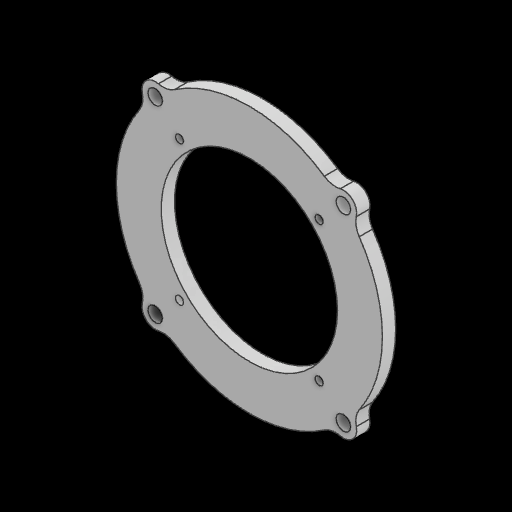
# Autodesk Inventor part: CimCoderMount
Saved by Autodesk Inventor 2025.2 (Build 292293000, 293)
## iProperties
Created: 2026-01-26
Part Number: CimCoderMount
Material: Generic
Document SubType Name: Sheet Metal
Designer: valer
Density: 1 g/cm^3
Appearance: Default
Sheet Metal Rule: Default
Author: valer
Autodesk Inventor part; units mm, degrees
ref_plane "YZ Plane" through (0, 0, 0) normal (1, 0, 0) x (0, 1, 0)
ref_plane "XZ Plane" through (0, 0, 0) normal (0, 1, 0) x (-1, 0, 0)
ref_plane "XY Plane" through (0, 0, 0) normal (0, 0, 1) x (1, 0, 0)
sketch "Base" plane through (0, 0, 0) normal (0, 0, 1) x (1, 0, 0)
  line L0 (-56, 0) -> (56, 0)
  line L1 (0, -56) -> (0, 56) construction
  circle A0 centre (0, 0) radius 40
  line L2 (0, 0) -> (28.2843, 28.2843) construction
  circle A1 centre (28.2843, 28.2843) radius 2.2
  circle A2 centre (-28.2843, 28.2843) radius 2.2
  circle A3 centre (28.2843, -28.2843) radius 2.2
  circle A4 centre (-28.2843, -28.2843) radius 2.2
  circle A5 centre (28.2843, 28.2843) radius 4
  circle A6 centre (-28.2843, 28.2843) radius 4
  circle A7 centre (28.2843, -28.2843) radius 4
  circle A8 centre (-28.2843, -28.2843) radius 4
  circle A9 centre (0, 0) radius 12.2174 construction
  spline S0 degree 3 number of poles 906
  spline S1 degree 3 number of poles 906
  spline S2 degree 3 number of poles 906
  spline S3 degree 3 number of poles 906
  spline S4 degree 2 poles (23.8703, -1.5488) (24.7501, -1.6971) (25.0615, -2.5332) (25.373, -3.3693) (24.8047, -4.057) (24.2364, -4.7448) (23.3566, -4.5965) (22.4768, -4.4482) (22.1653, -3.6122) (21.8538, -2.7761) (22.4222, -2.0883) (22.9905, -1.4006) (23.8703, -1.5488) (24.7501, -1.6971) (25.0615, -2.5332) (25.373, -3.3693) (24.8047, -4.057) (24.2364, -4.7448) (23.3566, -4.5965) (22.4768, -4.4482) (22.1653, -3.6122) (21.8538, -2.7761) (22.4222, -2.0883) (22.9905, -1.4006) (23.8703, -1.5488) (24.7501, -1.6971) (25.0615, -2.5332) (25.373, -3.3693) (24.8047, -4.057) (24.2364, -4.7448) (23.3566, -4.5965) (22.4768, -4.4482) (22.1653, -3.6122) (21.8538, -2.7761) (22.4222, -2.0883) (22.9905, -1.4006) (23.8703, -1.5488) (24.7501, -1.6971) (25.0615, -2.5332) (25.373, -3.3693) (24.8047, -4.057) (24.2364, -4.7448) (23.3566, -4.5965) (22.4768, -4.4482) (22.1653, -3.6122) (21.8538, -2.7761) (22.4222, -2.0883) (22.9905, -1.4006) (23.8703, -1.5488) (24.7501, -1.6971) (25.0615, -2.5332) (25.373, -3.3693) (24.8047, -4.057) (24.2364, -4.7448) (23.3566, -4.5965) (22.4768, -4.4482) (22.1653, -3.6122) (21.8538, -2.7761) (22.4222, -2.0883) (22.9905, -1.4006) (23.8703, -1.5488) (24.7501, -1.6971) (25.0615, -2.5332) (25.373, -3.3693) (24.8047, -4.057) (24.2364, -4.7448) (23.3566, -4.5965) (22.4768, -4.4482) (22.1653, -3.6122) (21.8538, -2.7761) (22.4222, -2.0883) (22.9905, -1.4006) (23.8703, -1.5488) (24.7501, -1.6971) (25.0615, -2.5332) (25.373, -3.3693) (24.8047, -4.057) (24.2364, -4.7448) (23.3566, -4.5965) (22.4768, -4.4482) (22.1653, -3.6122) (21.8538, -2.7761) (22.4222, -2.0883) (22.9905, -1.4006) (23.8703, -1.5488) (24.7501, -1.6971) (25.0615, -2.5332) (25.373, -3.3693) (24.8047, -4.057) (24.2364, -4.7448) (23.3566, -4.5965) (22.4768, -4.4482) (22.1653, -3.6122) (21.8538, -2.7761) (22.4222, -2.0883) (22.9905, -1.4006) (23.8703, -1.5488) (24.7501, -1.6971) (25.0615, -2.5332) (25.373, -3.3693) (24.8047, -4.057) (24.2364, -4.7448) (23.3566, -4.5965) (22.4768, -4.4482) (22.1653, -3.6122) (21.8538, -2.7761) (22.4222, -2.0883) (22.9905, -1.4006) (23.8703, -1.5488) (24.7501, -1.6971) (25.0615, -2.5332) (25.373, -3.3693) (24.8047, -4.057) (24.2364, -4.7448) (23.3566, -4.5965) (22.4768, -4.4482) (22.1653, -3.6122) (21.8538, -2.7761) (22.4222, -2.0883) (22.9905, -1.4006) (23.8703, -1.5488) (24.7501, -1.6971) (25.0615, -2.5332) (25.373, -3.3693) (24.8047, -4.057) (24.2364, -4.7448) (23.3566, -4.5965) (22.4768, -4.4482) (22.1653, -3.6122) (21.8538, -2.7761) (22.4222, -2.0883) (22.9905, -1.4006) (23.8703, -1.5488) (24.7501, -1.6971) (25.0615, -2.5332) (25.373, -3.3693) (24.8047, -4.057) (24.2364, -4.7448) (23.3566, -4.5965) (22.4768, -4.4482) (22.1653, -3.6122) (21.8538, -2.7761) (22.4222, -2.0883) (22.9905, -1.4006) (23.8703, -1.5488) (24.7501, -1.6971) (25.0615, -2.5332) (25.373, -3.3693) (24.8047, -4.057) (24.2364, -4.7448) (23.3566, -4.5965) (22.4768, -4.4482) (22.1653, -3.6122) (21.8538, -2.7761) (22.4222, -2.0883) (22.9905, -1.4006) (23.8703, -1.5488) (24.7501, -1.6971) (25.0615, -2.5332) (25.373, -3.3693) (24.8047, -4.057) (24.2364, -4.7448) (23.3566, -4.5965) (22.4768, -4.4482) (22.1653, -3.6122) (21.8538, -2.7761) (22.4222, -2.0883) (22.9905, -1.4006) (23.8703, -1.5488) (24.7501, -1.6971) (25.0615, -2.5332) (25.373, -3.3693) (24.8047, -4.057) (24.2364, -4.7448) (23.3566, -4.5965) (22.4768, -4.4482) (22.1653, -3.6122) (21.8538, -2.7761) (22.4222, -2.0883) (22.9905, -1.4006) (23.8703, -1.5488) (24.7501, -1.6971) (25.0615, -2.5332) (25.373, -3.3693) (24.8047, -4.057) (24.2364, -4.7448) (23.3566, -4.5965) (22.4768, -4.4482) (22.1653, -3.6122) (21.8538, -2.7761) (22.4222, -2.0883) (22.9905, -1.4006) (23.8703, -1.5488) (24.7501, -1.6971) (25.0615, -2.5332) (25.373, -3.3693) (24.8047, -4.057) (24.2364, -4.7448) (23.3566, -4.5965) (22.4768, -4.4482) (22.1653, -3.6122) (21.8538, -2.7761) (22.4222, -2.0883) (22.9905, -1.4006) (23.8703, -1.5488) (24.7501, -1.6971) (25.0615, -2.5332) (25.373, -3.3693) (24.8047, -4.057) (24.2364, -4.7448) (23.3566, -4.5965) (22.4768, -4.4482) (22.1653, -3.6122) (21.8538, -2.7761) (22.4222, -2.0883) (22.9905, -1.4006) (23.8703, -1.5488) (24.7501, -1.6971) (25.0615, -2.5332) (25.373, -3.3693) (24.8047, -4.057) (24.2364, -4.7448) (23.3566, -4.5965) (22.4768, -4.4482) (22.1653, -3.6122) (21.8538, -2.7761) (22.4222, -2.0883) (22.9905, -1.4006) (23.8703, -1.5488) (24.7501, -1.6971) (25.0615, -2.5332) (25.373, -3.3693) (24.8047, -4.057) (24.2364, -4.7448) (23.3566, -4.5965) (22.4768, -4.4482) (22.1653, -3.6122) (21.8538, -2.7761) (22.4222, -2.0883) (22.9905, -1.4006) (23.8703, -1.5488) (24.7501, -1.6971) (25.0615, -2.5332) (25.373, -3.3693) (24.8047, -4.057) (24.2364, -4.7448) (23.3566, -4.5965) (22.4768, -4.4482) (22.1653, -3.6122) (21.8538, -2.7761) (22.4222, -2.0883) (22.9905, -1.4006) (23.8703, -1.5488) (24.7501, -1.6971) (25.0615, -2.5332) (25.373, -3.3693) (24.8047, -4.057) (24.2364, -4.7448) (23.3566, -4.5965) (22.4768, -4.4482) (22.1653, -3.6122) (21.8538, -2.7761) (22.4222, -2.0883) (22.9905, -1.4006) (23.8703, -1.5488) (24.7501, -1.6971) (25.0615, -2.5332) (25.373, -3.3693) (24.8047, -4.057) (24.2364, -4.7448) (23.3566, -4.5965) (22.4768, -4.4482) (22.1653, -3.6122) (21.8538, -2.7761) (22.4222, -2.0883) (22.9905, -1.4006) (23.8703, -1.5488) (24.7501, -1.6971) (25.0615, -2.5332) (25.373, -3.3693) (24.8047, -4.057) (24.2364, -4.7448) (23.3566, -4.5965) (22.4768, -4.4482) (22.1653, -3.6122) (21.8538, -2.7761) (22.4222, -2.0883) (22.9905, -1.4006) (23.8703, -1.5488) (24.7501, -1.6971) (25.0615, -2.5332) (25.373, -3.3693) (24.8047, -4.057) (24.2364, -4.7448) (23.3566, -4.5965) (22.4768, -4.4482) (22.1653, -3.6122) (21.8538, -2.7761) (22.4222, -2.0883) (22.9905, -1.4006) (23.8703, -1.5488) (24.7501, -1.6971) (25.0615, -2.5332) (25.373, -3.3693) (24.8047, -4.057) (24.2364, -4.7448) (23.3566, -4.5965) (22.4768, -4.4482) (22.1653, -3.6122) (21.8538, -2.7761) (22.4222, -2.0883) (22.9905, -1.4006) (23.8703, -1.5488) (24.7501, -1.6971) (25.0615, -2.5332) (25.373, -3.3693) (24.8047, -4.057) (24.2364, -4.7448) (23.3566, -4.5965) (22.4768, -4.4482) (22.1653, -3.6122) (21.8538, -2.7761) (22.4222, -2.0883) (22.9905, -1.4006) (23.8703, -1.5488) (24.7501, -1.6971) (25.0615, -2.5332) (25.373, -3.3693) (24.8047, -4.057) (24.2364, -4.7448) (23.3566, -4.5965) (22.4768, -4.4482) (22.1653, -3.6122) (21.8538, -2.7761) (22.4222, -2.0883) (22.9905, -1.4006) (23.8703, -1.5488) (24.7501, -1.6971) (25.0615, -2.5332) (25.1147, -2.6758) (25.139, -2.8261) knots 0.016667 0.016667 0.016667 0.022222 0.022222 0.027778 0.027778 0.033333 0.033333 0.038889 0.038889 0.044444 0.044444 0.05 0.05 0.055556 0.055556 0.061111 0.061111 0.066667 0.066667 0.072222 0.072222 0.077778 0.077778 0.083333 0.083333 0.088889 0.088889 0.094444 0.094444 0.1 0.1 0.105556 0.105556 0.111111 0.111111 0.116667 0.116667 0.122222 0.122222 0.127778 0.127778 0.133333 0.133333 0.138889 0.138889 0.144444 0.144444 0.15 0.15 0.155556 0.155556 0.161111 0.161111 0.166667 0.166667 0.172222 0.172222 0.177778 0.177778 0.183333 0.183333 0.188889 0.188889 0.194444 0.194444 0.2 0.2 0.205556 0.205556 0.211111 0.211111 0.216667 0.216667 0.222222 0.222222 0.227778 0.227778 0.233333 0.233333 0.238889 0.238889 0.244444 0.244444 0.25 0.25 0.255556 0.255556 0.261111 0.261111 0.266667 0.266667 0.272222 0.272222 0.277778 0.277778 0.283333 0.283333 0.288889 0.288889 0.294444 0.294444 0.3 0.3 0.305556 0.305556 0.311111 0.311111 0.316667 0.316667 0.322222 0.322222 0.327778 0.327778 0.333333 0.333333 0.338889 0.338889 0.344444 0.344444 0.35 0.35 0.355556 0.355556 0.361111 0.361111 0.366667 0.366667 0.372222 0.372222 0.377778 0.377778 0.383333 0.383333 0.388889 0.388889 0.394444 0.394444 0.4 0.4 0.405556 0.405556 0.411111 0.411111 0.416667 0.416667 0.422222 0.422222 0.427778 0.427778 0.433333 0.433333 0.438889 0.438889 0.444444 0.444444 0.45 0.45 0.455556 0.455556 0.461111 0.461111 0.466667 0.466667 0.472222 0.472222 0.477778 0.477778 0.483333 0.483333 0.488889 0.488889 0.494444 0.494444 0.5 0.5 0.505556 0.505556 0.511111 0.511111 0.516667 0.516667 0.522222 0.522222 0.527778 0.527778 0.533333 0.533333 0.538889 0.538889 0.544444 0.544444 0.55 0.55 0.555556 0.555556 0.561111 0.561111 0.566667 0.566667 0.572222 0.572222 0.577778 0.577778 0.583333 0.583333 0.588889 0.588889 0.594444 0.594444 0.6 0.6 0.605556 0.605556 0.611111 0.611111 0.616667 0.616667 0.622222 0.622222 0.627778 0.627778 0.633333 0.633333 0.638889 0.638889 0.644444 0.644444 0.65 0.65 0.655556 0.655556 0.661111 0.661111 0.666667 0.666667 0.672222 0.672222 0.677778 0.677778 0.683333 0.683333 0.688889 0.688889 0.694444 0.694444 0.7 0.7 0.705556 0.705556 0.711111 0.711111 0.716667 0.716667 0.722222 0.722222 0.727778 0.727778 0.733333 0.733333 0.738889 0.738889 0.744444 0.744444 0.75 0.75 0.755556 0.755556 0.761111 0.761111 0.766667 0.766667 0.772222 0.772222 0.777778 0.777778 0.783333 0.783333 0.788889 0.788889 0.794444 0.794444 0.8 0.8 0.805556 0.805556 0.811111 0.811111 0.816667 0.816667 0.822222 0.822222 0.827778 0.827778 0.833333 0.833333 0.838889 0.838889 0.844444 0.844444 0.85 0.85 0.855556 0.855556 0.861111 0.861111 0.866667 0.866667 0.872222 0.872222 0.877778 0.877778 0.883333 0.883333 0.888889 0.888889 0.894444 0.894444 0.9 0.9 0.905556 0.905556 0.911111 0.911111 0.916667 0.916667 0.922222 0.922222 0.927778 0.927778 0.933333 0.933333 0.938889 0.938889 0.944444 0.944444 0.95 0.95 0.955556 0.955556 0.956622 0.956622 0.956622 weights 1 0.866025 1 0.866025 1 0.866025 1 0.866025 1 0.866025 1 0.866025 1 0.866025 1 0.866025 1 0.866025 1 0.866025 1 0.866025 1 0.866025 1 0.866025 1 0.866025 1 0.866025 1 0.866025 1 0.866025 1 0.866025 1 0.866025 1 0.866025 1 0.866025 1 0.866025 1 0.866025 1 0.866025 1 0.866025 1 0.866025 1 0.866025 1 0.866025 1 0.866025 1 0.866025 1 0.866025 1 0.866025 1 0.866025 1 0.866025 1 0.866025 1 0.866025 1 0.866025 1 0.866025 1 0.866025 1 0.866025 1 0.866025 1 0.866025 1 0.866025 1 0.866025 1 0.866025 1 0.866025 1 0.866025 1 0.866025 1 0.866025 1 0.866025 1 0.866025 1 0.866025 1 0.866025 1 0.866025 1 0.866025 1 0.866025 1 0.866025 1 0.866025 1 0.866025 1 0.866025 1 0.866025 1 0.866025 1 0.866025 1 0.866025 1 0.866025 1 0.866025 1 0.866025 1 0.866025 1 0.866025 1 0.866025 1 0.866025 1 0.866025 1 0.866025 1 0.866025 1 0.866025 1 0.866025 1 0.866025 1 0.866025 1 0.866025 1 0.866025 1 0.866025 1 0.866025 1 0.866025 1 0.866025 1 0.866025 1 0.866025 1 0.866025 1 0.866025 1 0.866025 1 0.866025 1 0.866025 1 0.866025 1 0.866025 1 0.866025 1 0.866025 1 0.866025 1 0.866025 1 0.866025 1 0.866025 1 0.866025 1 0.866025 1 0.866025 1 0.866025 1 0.866025 1 0.866025 1 0.866025 1 0.866025 1 0.866025 1 0.866025 1 0.866025 1 0.866025 1 0.866025 1 0.866025 1 0.866025 1 0.866025 1 0.866025 1 0.866025 1 0.866025 1 0.866025 1 0.866025 1 0.866025 1 0.866025 1 0.866025 1 0.866025 1 0.866025 1 0.866025 1 0.866025 1 0.866025 1 0.866025 1 0.866025 1 0.866025 1 0.866025 1 0.866025 1 0.866025 1 0.866025 1 0.866025 1 0.866025 1 0.866025 1 0.866025 1 0.866025 1 0.866025 1 0.866025 1 0.866025 1 0.866025 1 0.866025 1 0.866025 1 0.866025 1 0.866025 1 0.866025 1 0.866025 1 0.866025 1 0.866025 1 0.866025 1 0.866025 1 0.866025 1 0.866025 1 0.866025 1 0.866025 1 0.866025 1 0.866025 1 0.866025 1 0.866025 1 0.866025 1 0.866025 1 0.866025 1 0.866025 1 0.866025 1 0.866025 1 0.866025 1 0.974286 0.958443
  arc A10 (7.6354, -22.3136) -> (7.8387, -21.1617) centre (9.1457, -21.9862) ccw
  circle A11 centre (0, 0) radius 26.5
  point P0 (0, 0)
  point P1 (25.318, 30.9677)
  point P2 (-25.318, 30.9677)
  point P3 (-30.9677, 25.318)
  point P4 (-40, 0)
  point P5 (40, 0)
  point P6 (30.9677, 25.318)
  point P7 (30.9677, -25.318)
  point P8 (-30.9677, -25.318)
  point P9 (-25.318, -30.9677)
  point P10 (25.318, -30.9677)
  point P11 (-29.7965, 26.6864)
  point P12 (-26.6864, 29.7965)
  point P13 (-26.6864, -29.7965)
  point P14 (-29.7965, -26.6864)
extrude "Plate1" add sketch "Base" along normal blind 4 contours A11 L0 A0 A6 A5 | L0 A0 A7 A8 A11 | A5 A0 A1 | A0 A1 A5 | A7 A0 A3 | A0 A3 A7 | A6 A0 A2 | A0 A2 A6 | A8 A0 A4 | A0 A4 A8
fillet "FilletsFeature" radius 6 8 edges at (-30.9677, 25.318, 2) (-30.9677, -25.318, 2) (-25.318, -30.9677, 2) (25.318, -30.9677, 2) (30.9677, -25.318, 2) (30.9677, 25.318, 2) (25.318, 30.9677, 2) (-25.318, 30.9677, 2)
sketch "WheelEncoderMount" plane through (0, 0, 4) normal (0, 0, 1) x (1, 0, 0)
  circle A0 centre (-20.9919, -21) radius 1.25 projected
  circle A1 centre (-20.9919, 21) radius 1.25 projected
  circle A2 centre (21.0081, -21) radius 1.25 projected
  circle A3 centre (21.0081, 21) radius 1.25 projected
  circle A4 centre (-20.9919, -21) radius 1.25 projected
  circle A5 centre (-20.9919, 21) radius 1.25 projected
  constraints: 4 coincident
hole "EncoderMountHolesFeature" at (-20.9919, -21, 4) at (-20.9919, 21, 4) at (21.0081, 21, 4) at (21.0081, -21, 4) direction (0, 0, -1) diameter 2.45 end through all
equation "\"d48\" = Thickness"
equation "\"d28\" = Thickness"
equation "\"BendRadius\" = Thickness"
equation "\"BendReliefWidth\" = Thickness"
equation "\"BendReliefDepth\" = 0.5 * Thickness"
equation "\"CornerReliefSize\" = 4 * Thickness"
equation "\"MinimumRemnant\" = 2 * Thickness"
equation "\"TransitionRadius\" = BendRadius"
equation "\"JacobiRadiusSize\" = BendRadius"
equation "\"GapSize\" = Thickness"
equation "\"Thickness\" = 4"
body "Solid2"
